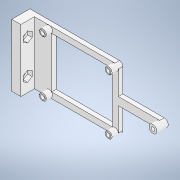
# Autodesk Inventor part: Support_Raspberry
Saved by Autodesk Inventor 2022 (Build 260153000, 153)
## iProperties
Created: 2021-12-07
Part Number: Support_Raspberry
Material: Générique
Document SubType Name: Modeling
Designer: utilisateur
Density: 1 g/cm^3
Appearance: Par défaut(1)
Author: utilisateur
Autodesk Inventor part; units mm, degrees
ref_plane "YZ Plane" through (0, 0, 0) normal (1, 0, 0) x (0, 1, 0)
ref_plane "XZ Plane" through (0, 0, 0) normal (0, 1, 0) x (-1, 0, 0)
ref_plane "XY Plane" through (0, 0, 0) normal (0, 0, 1) x (1, 0, 0)
sketch "Esquisse1" plane through (0, 0, 0) normal (0, 0, 1) x (1, 0, 0)
  line L0 (-29, 24.5) -> (29, 24.5) construction
  line L1 (29, 24.5) -> (29, -24.5) construction
  line L2 (29, -24.5) -> (-29, -24.5) construction
  line L3 (-29, -24.5) -> (-29, 24.5) construction
  line L4 (-29, 24.5) -> (29, -24.5) construction
  line L5 (29, 24.5) -> (-29, -24.5) construction
  circle A0 centre (29, 24.5) radius 1.65
  circle A1 centre (-29, 24.5) radius 1.65
  circle A2 centre (-29, -24.5) radius 1.65
  circle A3 centre (29, -24.5) radius 1.65
  circle A4 centre (29, 24.5) radius 3
  circle A5 centre (-29, 24.5) radius 3
  circle A6 centre (-29, -24.5) radius 3
  circle A7 centre (29, -24.5) radius 3
  line L6 (-42, -27.5) -> (-32, -27.5)
  line L7 (-32, -27.5) -> (-32, 27.5)
  line L8 (-32, 27.5) -> (-42, 27.5)
  line L9 (-42, 27.5) -> (-42, -27.5)
  line L10 (-42, -27.5) -> (-32, 27.5) construction
  line L11 (-32, -27.5) -> (-42, 27.5) construction
  line L12 (-50, -27.5) -> (-42, -27.5)
  line L13 (-42, -27.5) -> (-42, 27.5)
  line L14 (-42, 27.5) -> (-50, 27.5)
  line L15 (-50, 27.5) -> (-50, -27.5)
  line L16 (-50, -27.5) -> (-42, 27.5) construction
  line L17 (-42, -27.5) -> (-50, 27.5) construction
  line L18 (-74.4, 0) -> (96.4, 0) projected
  line L19 (-32, -27.5) -> (32, -27.5)
  line L20 (32, -27.5) -> (32, 27.5)
  line L21 (32, 27.5) -> (-32, 27.5)
  line L22 (-32, 27.5) -> (-32, -27.5)
  line L23 (-32, -27.5) -> (32, 27.5) construction
  line L24 (32, -27.5) -> (-32, 27.5) construction
  line L25 (26.8787, 22.3787) -> (-26.8787, 22.3787)
  line L26 (-26.8787, 22.3787) -> (-26.8787, -22.3787)
  line L27 (-26.8787, -22.3787) -> (26.8787, -22.3787)
  line L28 (26.8787, -22.3787) -> (26.8787, 22.3787)
  line L29 (26.8787, 22.3787) -> (-26.8787, -22.3787) construction
  line L30 (-26.8787, 22.3787) -> (26.8787, -22.3787) construction
  line L31 (26.8787, 0) -> (32, 0) construction
  line L32 (0, -22.3787) -> (0, -27.5) construction
  line L33 (72, -3.5) -> (32, -3.5)
  line L34 (32, -3.5) -> (32, 3.5)
  line L35 (32, 3.5) -> (72, 3.5)
  line L36 (72, 3.5) -> (72, -3.5)
  line L37 (72, -3.5) -> (32, 3.5) construction
  line L38 (32, -3.5) -> (72, 3.5) construction
  circle A8 centre (68.5, 0) radius 3.5
  circle A9 centre (68.5, 0) radius 1.65
  point P0 (0, 0)
  point P1 (-29, 0)
  point P2 (0, -24.5)
  point P3 (-37, 0)
  point P4 (-46, 0)
  point P5 (-32, 0)
  point P6 (-29, -27.5)
  point P7 (29, -27.5)
  point P8 (32, -24.5)
  point P9 (-29, 27.5)
  point P10 (-32, 24.5)
  point P11 (-32, -24.5)
  point P12 (32, 24.5)
  point P13 (29, 27.5)
  point P14 (52, 0)
  point P15 (68.5, -3.5)
  point P16 (68.5, 3.5)
  dimension "d3" = 6
  dimension "d0" = 49
  dimension "d1" = 58
  dimension "d2" = 3.3
  dimension "d32" = 10
  dimension "d33" = 8
  dimension "d49" = 7
  dimension "d50" = 40
  constraints: 76 end point, 20 midpoint, 12 parallel, 9 centre point, 7 horizontal, 7 perpendicular, 6 equal radius, 5 coincident, 5 point on line, 2 tangent, 1 collinear, 1 vertical, 4 other
  measures "d0" distance of L0.end L1.end
  measures "d1" distance of L0.start L0.end
  measures "d2" diameter of A1
  measures "d32" distance between parallel lines of L9 L7
  measures "d33" distance between parallel lines of L9 L15
  measures "d49" distance between parallel lines of L33 L35
  measures "d50" distance between parallel lines of L20 L36
extrude "Extrusion1" add sketch "Esquisse1" against normal blind 4 contours A4 | L25 A5 L21 A4 | A4 L20 L18 L28 | A5 | L26 L18 L7 A5 | L18 L20 A7 L28 | L35 A8 L18 L20 | A5 L7 L21 | L7 L18 L9 L8 | L26 A6 L7 L18 | L18 A8 L33 L20 | A7 | A7 L19 A6 L27 | A8 L18 A9 | L7 L6 L9 L18 | A6 | L18 A9 A8 | L9 L18 L15 L14 | A6 L19 L7 | L9 L12 L15 L18
extrude "Extrusion10" add sketch "Esquisse1" along normal blind 12 contours L9 L18 L15 L14 | L9 L12 L15 L18
extrude "Extrusion11" add sketch "Esquisse1" along normal blind 6 contours A4 | A5 | A7 | A8 L18 A9 | A6 | L18 A9 A8
sketch "Esquisse13" plane through (-42, -27.5, 0) normal (1, 0, 0) x (0, 0, -1)
  line L0 (0, 55) -> (0, 0) projected
  line L1 (0, 55) -> (-12, 55) projected
  line L2 (-12, 0) -> (-12, 55) projected
  line L3 (0, 0) -> (-12, 0) projected
  line L4 (0, 0) -> (-12, 0) projected
  line L5 (-6, 0) -> (-6, 12.5)
  line L6 (-6, 12.5) -> (-6, 42.5) construction
  line L7 (-6, 42.5) -> (-6, 55)
  line L8 (0, 55) -> (-12, 55) projected
  circle A0 centre (-6, 12.5) radius 2.1
  circle A1 centre (-6, 42.5) radius 2.1
  line L9 (-2, 14.8094) -> (-2, 10.1906)
  line L10 (-2, 10.1906) -> (-6, 7.8812)
  line L11 (-6, 7.8812) -> (-10, 10.1906)
  line L12 (-10, 10.1906) -> (-10, 14.8094)
  line L13 (-10, 14.8094) -> (-6, 17.1188)
  line L14 (-6, 17.1188) -> (-2, 14.8094)
  line L15 (-6, 37.8812) -> (-10, 40.1906)
  line L16 (-10, 40.1906) -> (-10, 44.8094)
  line L17 (-10, 44.8094) -> (-6, 47.1188)
  line L18 (-6, 47.1188) -> (-2, 44.8094)
  line L19 (-2, 44.8094) -> (-2, 40.1906)
  line L20 (-2, 40.1906) -> (-6, 37.8812)
  point P0 (-10, 42.5)
  dimension "d38" = 4.2
  dimension "d39" = 8
  dimension "d41" = 30
  constraints: 30 end point, 4 coincident, 3 midpoint, 3 vertical, 2 centre point, 2 collinear, 1 equal radius, 1 point on line, 26 other
  measures "d38" diameter of A0
  measures "d39" distance between parallel lines of L9 L12
  measures "d41" distance of L5.end L6.end
extrude "Extrusion12" cut sketch "Esquisse13" against normal through all contours A1 | A0
extrude "Extrusion13" cut sketch "Esquisse13" against normal blind 4 contours L18 L19 L20 L15 L16 L17 | L11 L12 L13 L14 L9 L10
chamfer "Chanfrein2" distance 0.5 angle 45 4 edges at (-32, -24.5, 6) (26, -24.5, 6) (26, 24.5, 6) (-32, 24.5, 6)
